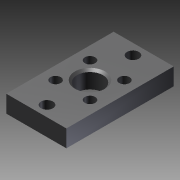
# Autodesk Inventor part: 537245 FNC-12---(F)
Saved by Autodesk Inventor 2011 SP1 (Build 150282100, 282)
## iProperties
Created: 2018-05-28
Part Number: 537245 FNC-12---(F)
Catalog Web Link: www.cadenas.de
Description: FNC-(F)-Flange mounting
Vendor: FESTO
Document SubType Name: Modeling
Designer: psAdmin
Manufacturer: FESTO
Mass: 8.67274 g
Surface Area: 48.2289 cm^2
Volume: 8.67274 cm^3
Density: 1 g/cm^3
Category: PARTsolutions
Company: FESTO
Title: 537245 FNC-12
Author: Cadenas PARTsolutions
Comments: Flange mounting
PSOL_IDENT_0: {$CADENAS_DATA\23d-libs\festo\parts\f\fnc\fnc.prj},175 {VTYP=3D},{NB=537245 FNC-12---(F)},{LINA=5372
PSOL_IDENT_1: 45 FNC-12},{NN=FNC-(F)},{DATE=13.11.2017 12:35:20},{GEOMDATE=13.11.2017 12:34:23},{VERSION=},{LINEID=
PSOL_IDENT_2: 80},{LINESUBID=-1},{WBVAR=}  {NB=537245 FNC-12---(F)},{LINA=537245 FNC-12},{KT=DUMMY},{TNR=537245},{
PSOL_IDENT_3: TYP=FNC-12},{VERS=1},{D1=12.000},{D2=4.800},{D3=8.000},{E=28.000},{F=1.000},{FB=5.500},{MF=8.000},{R=
PSOL_IDENT_4: 0.000},{T=3.000},{TF=40.000},{TG1=16.000},{UF=50.000},{ZZ=0},{DK=12},{D6912D=4.000},{D6912L=16.000}
NN: FNC-(F)
NT: Flange mounting
NB: 537245 FNC-12---(F)
NBSYN: $TNR. $TYP.---(F)
LINA: 537245 FNC-12
TNR: 537245
TYP: FNC-12
D1: 12.000
D2: 4.800
D3: 8.000
E: 28.000
F: 1.000
FB: 5.500
MF: 8.000
R: 0.000
T: 3.000
TF: 40.000
TG1: 16.000
UF: 50.000
SUPPLIER: FESTO
ARTICLENO: 537245 FNC-12---(F)
BOMINFO: 537245 FNC-12
CREATOR: CADENAS GmbH
Autodesk Inventor part; units mm, degrees
sketch "Skizze_1" plane through (0, 0, 0) normal (0, 0, 1) x (1, 0, 0)
  line L0 (-14, 25) -> (-14, -25)
  line L1 (-14, -25) -> (14, -25)
  line L2 (14, -25) -> (14, 25)
  line L3 (14, 25) -> (-14, 25)
  circle A0 centre (0, 20) radius 2.75
  circle A1 centre (0, -20) radius 2.75
  constraints: 8 end point, 2 centre point
extrude "Extrusion1" add sketch "Skizze_1" along normal blind 8
sketch "Skizze_2_ALT_Drilling_1" plane through (0, 0, 0) normal (1, 0, 0) x (0, 1, 0)
  line L0 (0, 0) -> (0, 8)
  line L1 (0, 8) -> (7, 8)
  line L2 (7, 8) -> (6, 7)
  line L3 (6, 7) -> (6, 0)
  line L4 (6, 0) -> (0, 0)
  line L5 (0, 0) -> (0, 8)
  constraints: 12 end point
revolve "Revolution1" cut sketch "Skizze_2_ALT_Drilling_1" angle 360 about axis through (0, 0, 0) along (0, 0, -1)
sketch "Skizze_3_ALT_Drilling_2" plane through (8, 0, 0) normal (1, 0, 0) x (0, 0, -1)
  line L0 (0, 8) -> (-8, 8)
  line L1 (-8, 8) -> (-8, 10.4)
  line L2 (-8, 10.4) -> (-5, 10.4)
  line L3 (-5, 10.4) -> (-5, 12)
  line L4 (-5, 12) -> (0, 12)
  line L5 (0, 12) -> (0, 8)
  line L6 (0, 8) -> (-8, 8)
  constraints: 14 end point
revolve "Revolution2" cut sketch "Skizze_3_ALT_Drilling_2" angle 360 about axis through (8, 8, 0) along (0, 0, -1)
sketch "Muster_1_SKETCH_1" plane through (-8, 0, 0) normal (1, 0, 0) x (0, 0, -1)
  line L0 (0, 8) -> (-8, 8)
  line L1 (-8, 8) -> (-8, 10.4)
  line L2 (-8, 10.4) -> (-5, 10.4)
  line L3 (-5, 10.4) -> (-5, 12)
  line L4 (-5, 12) -> (0, 12)
  line L5 (0, 12) -> (0, 8)
  line L6 (0, 8) -> (-8, 8)
  constraints: 14 end point
sketch "Muster_1_SKETCH_2" plane through (8, 0, 0) normal (1, 0, 0) x (0, 0, -1)
  line L0 (0, -8) -> (-8, -8)
  line L1 (-8, -8) -> (-8, -5.6)
  line L2 (-8, -5.6) -> (-5, -5.6)
  line L3 (-5, -5.6) -> (-5, -4)
  line L4 (-5, -4) -> (0, -4)
  line L5 (0, -4) -> (0, -8)
  line L6 (0, -8) -> (-8, -8)
  constraints: 14 end point
sketch "Muster_1_SKETCH_3" plane through (-8, 0, 0) normal (1, 0, 0) x (0, 0, -1)
  line L0 (0, -8) -> (-8, -8)
  line L1 (-8, -8) -> (-8, -5.6)
  line L2 (-8, -5.6) -> (-5, -5.6)
  line L3 (-5, -5.6) -> (-5, -4)
  line L4 (-5, -4) -> (0, -4)
  line L5 (0, -4) -> (0, -8)
  line L6 (0, -8) -> (-8, -8)
  constraints: 14 end point
revolve "Revolution3" cut sketch "Muster_1_SKETCH_1" angle 360 about axis through (-8, 8, 0) along (0, 0, -1)
revolve "Revolution4" cut sketch "Muster_1_SKETCH_2" angle 360 about axis through (8, -8, 0) along (0, 0, -1)
revolve "Revolution5" cut sketch "Muster_1_SKETCH_3" angle 360 about axis through (-8, -8, 0) along (0, 0, -1)
ref_plane "FDT_MOUNT_XY" through (0, 0, 8) normal (0, 0, 1) x (0, 1, 0)
ref_plane "FDT_MOUNT_YZ" through (0, 0, 8) normal (0, 1, 0) x (-1, 0, 0)
ref_plane "FDT_MOUNT_ZX" through (0, 0, 8) normal (-1, 0, 0) x (0, 0, 1)
ref_plane "FNC_1_XY" through (0, 0, 4) normal (0, 0, 1) x (1, 0, 0)
ref_plane "FNC_1_YZ" through (0, 0, 4) normal (1, 0, 0) x (0, 1, 0)
ref_plane "FNC_1_ZX" through (0, 0, 4) normal (0, 1, 0) x (0, 0, 1)
ref_plane "FNC_2_3_XY" through (0, 0, 8) normal (0, 0, 1) x (1, 0, 0)
ref_plane "FNC_2_3_YZ" through (0, 0, 8) normal (1, 0, 0) x (0, 1, 0)
ref_plane "FNC_2_3_ZX" through (0, 0, 8) normal (0, 1, 0) x (0, 0, 1)
ref_plane "FNC_Schraube_1_XY" through (-8, 8, 5) normal (0, 0, 1) x (1, 0, 0)
ref_plane "FNC_Schraube_1_YZ" through (-8, 8, 5) normal (1, 0, 0) x (0, 1, 0)
ref_plane "FNC_Schraube_1_ZX" through (-8, 8, 5) normal (0, 1, 0) x (0, 0, 1)
ref_plane "FNC_Schraube_2_XY" through (8, 8, 5) normal (0, 0, 1) x (1, 0, 0)
ref_plane "FNC_Schraube_2_YZ" through (8, 8, 5) normal (1, 0, 0) x (0, 1, 0)
ref_plane "FNC_Schraube_2_ZX" through (8, 8, 5) normal (0, 1, 0) x (0, 0, 1)
ref_plane "FNC_Schraube_3_XY" through (-8, -8, 5) normal (0, 0, 1) x (1, 0, 0)
ref_plane "FNC_Schraube_3_YZ" through (-8, -8, 5) normal (1, 0, 0) x (0, 1, 0)
ref_plane "FNC_Schraube_3_ZX" through (-8, -8, 5) normal (0, 1, 0) x (0, 0, 1)
ref_plane "FNC_Schraube_4_XY" through (8, -8, 5) normal (0, 0, 1) x (1, 0, 0)
ref_plane "FNC_Schraube_4_YZ" through (8, -8, 5) normal (1, 0, 0) x (0, 1, 0)
ref_plane "FNC_Schraube_4_ZX" through (8, -8, 5) normal (0, 1, 0) x (0, 0, 1)
ref_plane "P17_1_XY" through (0, 20, 8) normal (0, 0, 1) x (1, 0, 0)
ref_plane "P17_1_YZ" through (0, 20, 8) normal (1, 0, 0) x (0, 1, 0)
ref_plane "P17_1_ZX" through (0, 20, 8) normal (0, 1, 0) x (0, 0, 1)
ref_plane "P18_1_XY" through (0, -20, 8) normal (0, 0, 1) x (1, 0, 0)
ref_plane "P18_1_YZ" through (0, -20, 8) normal (1, 0, 0) x (0, 1, 0)
ref_plane "P18_1_ZX" through (0, -20, 8) normal (0, 1, 0) x (0, 0, 1)
body "Solid1"
